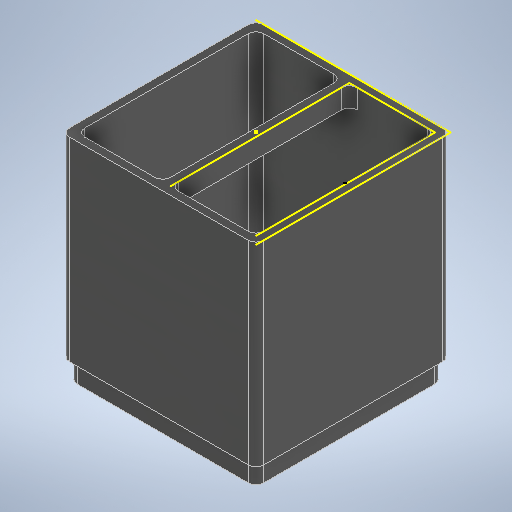
# Autodesk Inventor part: Część1
Saved by Autodesk Inventor 2025.2 (Build 292293000, 293)
## iProperties
Created: 2024-12-19
Part Number: Część1
Material: Ogólny
Document SubType Name: Sheet Metal
Designer: kamil
Density: 1 g/cm^3
Sheet Metal Rule: Domyślny_mm
Appearance: Ciemnoszara
Author: kamil
Autodesk Inventor part; units mm, degrees
ref_plane "YZ Plane" through (0, 0, 0) normal (1, 0, 0) x (0, 1, 0)
ref_plane "XZ Plane" through (0, 0, 0) normal (0, 1, 0) x (-1, 0, 0)
ref_plane "XY Plane" through (0, 0, 0) normal (0, 0, 1) x (1, 0, 0)
sketch "Szkic1" plane through (0, 0, 0) normal (0, 1, 0) x (-1, 0, 0)
  line L0 (-50, -50) -> (50, -50)
  line L1 (50, -50) -> (50, 50)
  line L2 (50, 50) -> (-50, 50)
  line L3 (-50, 50) -> (-50, -50)
  line L4 (-50, -50) -> (50, 50) construction
  line L5 (50, -50) -> (-50, 50) construction
  point P0 (0, 0)
  dimension "d0" = 100
  dimension "d1" = 100
  constraints: 12 end point, 2 midpoint, 2 parallel, 1 horizontal, 1 perpendicular
  measures "d0" distance of L2.end L1.end
  measures "d1" distance of L1.end L0.end
extrude "Wyciągnięcie proste1" add sketch "Szkic1" along normal blind 100
sketch "Szkic2" plane through (0, 100, 0) normal (0, 1, 0) x (1, 0, 0)
  line L0 (46, -46) -> (-46, -46)
  line L1 (-46, -46) -> (-46, 46)
  line L2 (-46, 46) -> (46, 46)
  line L3 (46, 46) -> (46, -46)
  line L4 (46, -46) -> (-46, 46) construction
  line L5 (-46, -46) -> (46, 46) construction
  point P0 (0, 0)
  dimension "d4" = 92
  dimension "d5" = 92
  constraints: 12 end point, 2 midpoint, 2 parallel, 1 horizontal, 1 perpendicular
  measures "d4" distance of L1.end L2.end
  measures "d5" distance of L0.end L1.end
extrude "Wyciągnięcie proste2" cut sketch "Szkic2" against normal blind 100
sketch "Szkic3" plane through (0, 0, 0) normal (0, -1, 0) x (1, 0, 0)
  line L0 (-48, -48) -> (48, -48)
  line L1 (48, -48) -> (48, 48)
  line L2 (48, 48) -> (-48, 48)
  line L3 (-48, 48) -> (-48, -48)
  line L4 (-48, -48) -> (48, 48) construction
  line L5 (48, -48) -> (-48, 48) construction
  line L6 (-46, -46) -> (46, -46)
  line L7 (46, -46) -> (46, 46)
  line L8 (46, 46) -> (-46, 46)
  line L9 (-46, 46) -> (-46, -46)
  line L10 (-46, -46) -> (46, 46) construction
  line L11 (46, -46) -> (-46, 46) construction
  point P0 (0, 0)
  dimension "d8" = 96
  dimension "d9" = 96
  dimension "d10" = 92
  dimension "d11" = 92
  constraints: 24 end point, 4 midpoint, 4 parallel, 2 horizontal, 2 perpendicular
  measures "d8" distance of L2.end L1.end
  measures "d9" distance of L1.end L0.end
  measures "d10" distance of L8.end L7.end
  measures "d11" distance of L7.end L6.end
extrude "Wyciągnięcie proste3" add sketch "Szkic3" along normal blind 10 contours L3 L2 L1 L0 | L9 L8 L7 L6
sketch "Szkic4" plane through (0, -10, 0) normal (0, -1, 0) x (1, 0, 0)
  line L0 (46, 46) -> (-46, 46)
  line L1 (-46, 46) -> (-46, -46)
  line L2 (-46, -46) -> (46, -46)
  line L3 (46, -46) -> (46, 46)
  line L4 (46, 46) -> (-46, -46) construction
  line L5 (-46, 46) -> (46, -46) construction
  point P0 (0, 0)
  dimension "d14" = 92
  dimension "d15" = 92
  constraints: 12 end point, 2 midpoint, 2 parallel, 1 horizontal, 1 perpendicular
  measures "d14" distance of L2.end L1.end
  measures "d15" distance of L1.end L0.end
extrude "Wyciągnięcie proste4" cut sketch "Szkic4" against normal blind 10
sketch "Szkic5" plane through (0, 100, 0) normal (0, 1, 0) x (1, 0, 0)
  line L0 (-2, 46) -> (2, 46)
  line L1 (2, 46) -> (2, -46)
  line L2 (2, -46) -> (-2, -46)
  line L3 (-2, -46) -> (-2, 46)
  line L4 (-2, 46) -> (2, -46) construction
  line L5 (2, 46) -> (-2, -46) construction
  point P0 (0, 0)
  dimension "d18" = 4
  dimension "d19" = 92
  constraints: 12 end point, 2 midpoint, 2 parallel, 1 horizontal, 1 perpendicular
  measures "d18" distance of L1.end L2.end
  measures "d19" distance of L0.end L1.end
extrude "Wyciągnięcie proste5" add sketch "Szkic5" against normal blind 10
sketch "Szkic6" plane through (0, 100, 0) normal (0, 1, 0) x (1, 0, 0)
  line L0 (46, 46) -> (46, -46) projected
  line L1 (2, 46) -> (46, 46) projected
  line L2 (50, 50) -> (-50, 50) projected
  line L3 (50, -50) -> (50, 50) projected
  line L4 (2, -46) -> (2, 46) projected
  point P0 (0, 0)
  point P1 (46, 0)
  constraints: 1 midpoint
fillet "Zaokrąglenie1" radius 4 16 edges at (2, 95, 46) (2, 95, -46) (-2, 95, -46) (-2, 95, 46) (50, 50, 50) (-50, 50, 50) (-50, 50, -50) (50, 50, -50) (46, 45, -46) (46, 45, 46) (-46, 45, 46) (-46, 45, -46) (-48, -5, 48) (48, -5, 48) (48, -5, -48) (-48, -5, -48)
equation "\"PromieńGięcia\" = Grubość"
equation "\"SzerokośćGięciaPodcięcia\" = Grubość"
equation "\"GłębokośćGięciaPodcięcia\" = 0.5 * Grubość"
equation "\"RozmiarPodcięciaNarożnika\" = 4 * Grubość"
equation "\"MinimalnaPozostałość\" = 2 * Grubość"
equation "\"PromieńPrzejścia\" = PromieńGięcia"
equation "\"Rozmiar_promienia_Jacobiego\" = PromieńGięcia"
equation "\"Wielk_odstępu\" = Grubość"
equation "\"Grubość\" = 0.5"
